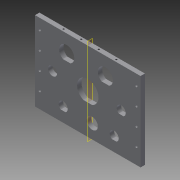
# Autodesk Inventor part: Yagi_Front_BackPlate
Saved by Autodesk Inventor 2014 (Build 180170000, 170)
## iProperties
Created: 2015-01-07
Part Number: Yagi_Front_BackPlate
Material: Generic
Document SubType Name: Modeling
Designer: Owner
Density: 1 g/cm^3
Appearance: Default
Author: Owner
Autodesk Inventor part; units mm, degrees
ref_plane "YZ Plane" through (0, 0, 0) normal (1, 0, 0) x (0, 1, 0)
ref_plane "XZ Plane" through (0, 0, 0) normal (0, 1, 0) x (-1, 0, 0)
ref_plane "XY Plane" through (0, 0, 0) normal (0, 0, 1) x (1, 0, 0)
sketch "Sketch1" plane through (0, 0, 0) normal (0, 0, 1) x (1, 0, 0)
  line L0 (-24.8346, -36.7982) -> (51.3654, -36.7982)
  line L1 (51.3654, -36.7982) -> (51.3654, -93.9482)
  line L2 (51.3654, -93.9482) -> (-24.8346, -93.9482)
  line L3 (-24.8346, -93.9482) -> (-24.8346, -36.7982)
  point P0 (0, 0)
  dimension "d0" = 76.2
  dimension "d1" = 57.15
  constraints: 8 end point, 2 parallel, 1 horizontal, 1 perpendicular
  measures "d0" distance of L0.start L0.end
  measures "d1" distance of L0.end L1.end
extrude "Extrusion1" add sketch "Sketch1" along normal blind 3.175
sketch "Sketch2" plane through (0, 0, 0) normal (0, 0, -1) x (-1, 0, 0)
  line L0 (24.8346, -93.9482) -> (24.8346, -36.7982) projected
  line L1 (-51.3654, -93.9482) -> (24.8346, -93.9482) projected
  circle A0 centre (-25.9654, -49.4982) radius 9.0932 construction
  arc A1 (-23.2263, -54.2226) -> (-28.7045, -54.2226) centre (-25.9654, -49.4982) ccw
  line L2 (-28.7045, -54.2226) -> (-23.2263, -54.2226)
  circle A2 centre (-13.2654, -65.3732) radius 10.3124 construction
  arc A3 (-10.0229, -72.409) -> (-16.5078, -72.409) centre (-13.2654, -65.3732) ccw
  line L3 (-16.5078, -72.409) -> (-10.0229, -72.409)
  circle A4 centre (1.9746, -49.4982) radius 9.0932 construction
  arc A5 (4.7137, -54.2226) -> (-0.7645, -54.2226) centre (1.9746, -49.4982) ccw
  line L4 (-0.7645, -54.2226) -> (4.7137, -54.2226)
  circle A6 centre (-16.4404, -83.7882) radius 4.1
  circle A7 centre (-16.4404, -83.7882) radius 5.25 construction
  line L5 (24.8346, -54.8925) -> (24.8346, -40.8771)
  line L6 (24.8346, -36.7982) -> (-51.3654, -36.7982) projected
  arc A8 (-30.5833, -86.5382) -> (-34.0474, -86.5382) centre (-32.3154, -83.7882) ccw
  line L7 (-30.5833, -86.5382) -> (-34.0474, -86.5382)
  circle A9 centre (-32.3154, -83.7882) radius 5.5 construction
  arc A10 (-35.6633, -64.9482) -> (-39.1274, -64.9482) centre (-37.3954, -62.1982) ccw
  line L8 (-35.6633, -64.9482) -> (-39.1274, -64.9482)
  circle A11 centre (-37.3954, -62.1982) radius 5.5 construction
  arc A12 (10.4026, -62.6232) -> (13.8667, -62.6232) centre (12.1346, -65.3732) ccw
  line L9 (10.4026, -62.6232) -> (13.8667, -62.6232)
  circle A13 centre (12.1346, -65.3732) radius 5.5 construction
  arc A14 (6.2467, -86.5382) -> (2.7826, -86.5382) centre (4.5146, -83.7882) ccw
  line L10 (6.2467, -86.5382) -> (2.7826, -86.5382)
  circle A15 centre (4.5146, -83.7882) radius 5.5 construction
  line L11 (-51.3654, -36.7982) -> (-51.3654, -93.9482) projected
  line L12 (-45.0154, -36.7982) -> (-45.0154, -93.9482) construction
  line L13 (12.1346, -93.9482) -> (12.1346, -36.7982) construction
  line L14 (-51.3654, -90.7732) -> (24.8346, -90.7732) construction
  line L15 (-51.3654, -39.9732) -> (24.8346, -39.9732) construction
  point P0 (0, 0)
  dimension "d28" = 18.1864
  dimension "d29" = 10.922
  dimension "d30" = 4.7244
  dimension "d31" = 20.6248
  dimension "d32" = 15.494
  dimension "d33" = 7.0358
  dimension "d34" = 18.1864
  dimension "d35" = 10.922
  dimension "d36" = 4.7244
  dimension "d41" = 8.2
  dimension "d42" = 10.5
  dimension "d49" = 6.5
  dimension "d53" = 2.75
  dimension "d54" = 11
  dimension "d55" = 0
  dimension "d56" = 6.5
  dimension "d57" = 2.75
  dimension "d58" = 11
  dimension "d59" = 0
  dimension "d60" = 6.5
  dimension "d61" = 2.75
  dimension "d62" = 11
  dimension "d63" = 0
  dimension "d64" = 6.5
  dimension "d65" = 2.75
  dimension "d66" = 11
  dimension "d67" = 0
  dimension "d68" = 6.35
  dimension "d69" = 12.7
  dimension "d70" = 3.175
  dimension "d71" = 3.175
  dimension "d72" = 28.575
  dimension "d73" = 31.75
  dimension "d75" = 25.4
  dimension "d76" = 0
  dimension "d79" = 44.45
  dimension "d80" = 10.16
  dimension "d81" = 38.1
  dimension "d82" = 28.575
  dimension "d83" = 7.62
  dimension "d139" = 10.16
  dimension "d140" = 10.16
  dimension "d141" = 12.7
  dimension "d142" = 12.7
  dimension "d143" = 10.16
  dimension "d144" = 28.575
  dimension "d145" = 7.62
  constraints: 24 end point, 16 centre point, 14 point on circle, 9 parallel, 9 point on line, 4 coincident, 2 perpendicular
  measures "d28" diameter of A0
  measures "d29" diameter of A1
  measures "d30" distance from line of L2 A1.centre
  measures "d31" diameter of A2
  measures "d32" diameter of A3
  measures "d33" distance from line of A3.centre L3
  measures "d34" diameter of A4
  measures "d35" diameter of A5
  measures "d36" distance from line of L4 A5.centre
  measures "d41" diameter of A6
  measures "d42" diameter of A7
  measures "d49" diameter of A8
  measures "d53" distance from line of L7 A8.centre
  measures "d54" diameter of A9
  measures "d55" distance of A9.centre A8.centre
  measures "d56" diameter of A10
  measures "d57" distance from line of L8 A10.centre
  measures "d58" diameter of A11
  measures "d59" distance of A11.centre A10.centre
  measures "d60" diameter of A12
  measures "d61" distance from line of L9 A12.centre
  measures "d62" diameter of A13
  measures "d63" distance of A13.centre A12.centre
  measures "d64" diameter of A14
  measures "d65" distance from line of L10 A14.centre
  measures "d66" diameter of A15
  measures "d67" distance of A15.centre A14.centre
  measures "d68" distance between parallel lines of L11 L12
  measures "d69" distance between parallel lines of L0 L13
  measures "d70" distance between parallel lines of L1 L14
  measures "d71" distance between parallel lines of L6 L15
  measures "d72" distance from line of L1 A13.centre
  measures "d73" distance from line of L1 A10.centre
  measures "d75" distance from line of L13 A2.centre
  measures "d76" distance from line of L13 A12.centre
  measures "d79" distance from line of L13 A8.centre
  measures "d80" distance from line of A4.centre L13
  measures "d81" distance from line of L13 A0.centre
  measures "d82" distance from line of L13 A6.centre
  measures "d83" distance from line of L13 A14.centre
  measures "d139" distance from line of L1 A14.centre
  measures "d140" distance from line of L1 A8.centre
  measures "d141" distance from line of L6 A0.centre
  measures "d142" distance from line of L6 A4.centre
  measures "d143" distance from line of L1 A6.centre
  measures "d144" distance from line of L6 A3.centre
  measures "d145" distance from line of L12 A10.centre
extrude "Extrusion2" cut sketch "Sketch2" against normal blind 6.35 contours L2 A1 | L3 A3 | L4 A5 | A6 | L7 A8 | L8 A10 | L9 A12 | L10 A14
sketch "Sketch6" plane through (0, 0, 0) normal (0, 0, -1) x (-1, 0, 0)
  point P0 (-48.1904, -44.4182)
hole "Hole5" at (48.1904, -44.4182, 0) direction (0, 0, 1) diameter 1.778 depth 3.175 countersink diameter 3.0226 countersink angle 82
pattern_linear "Rectangular Pattern2" count 4 spacing 12.7 along (0, -1, 0) of "Hole5"
ref_plane "Work Plane1" through (13.2654, -93.9482, 0) normal (1, 0, 0) x (0, 0, -1)
sketch "Sketch7" plane through (-24.8346, -36.7982, 0) normal (0, 1, 0) x (1, 0, 0)
  point P0 (57.15, -1.5875)
hole "Hole7" at (32.3154, -36.7982, 1.5875) direction (0, -1, 0) diameter 1.1811 depth 4.699 tip angle 120 thread size "0-80 UNF" class "2B" standard "ANSI Unified Screw Threads"
pattern_linear "Rectangular Pattern3" count 2 spacing 12.7 along (-1, 0, 0) of "Hole7"
sketch "Sketch8" plane through (-24.8346, -93.9482, 0) normal (0, -1, 0) x (1, 0, 0)
  point P0 (19.05, 1.5875)
hole "Hole9" at (-5.7846, -93.9482, 1.5875) direction (0, 1, 0) diameter 1.1811 depth 4.699 tip angle 120 thread size "0-80 UNF" class "2B" standard "ANSI Unified Screw Threads"
pattern_linear "Rectangular Pattern4" count 2 spacing 12.7 along (1, 0, 0) of "Hole9"
mirror "Mirror1" about plane through (13.2654, -93.9482, 0) normal (1, 0, 0) of "Hole5", "Rectangular Pattern2", "Hole7", "Rectangular Pattern3", "Hole9", "Rectangular Pattern4"
body "Solid1"
